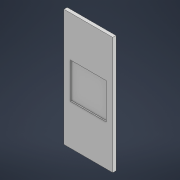
# Autodesk Inventor part: Shoulder_Cube_TestFit_V1
Saved by Autodesk Inventor 2022 (Build 260153000, 153)
## iProperties
Created: 2023-05-16
Part Number: Shoulder_Cube_TestFit_V1
Material: Generic
Document SubType Name: Modeling
Designer: Karl Spiteri
Density: 1 g/cm^3
Appearance: Default
Author: Karl Spiteri
Autodesk Inventor part; units mm, degrees
ref_plane "YZ Plane" through (0, 0, 0) normal (1, 0, 0) x (0, 1, 0)
ref_plane "XZ Plane" through (0, 0, 0) normal (0, 1, 0) x (-1, 0, 0)
ref_plane "XY Plane" through (0, 0, 0) normal (0, 0, 1) x (1, 0, 0)
sketch "Sketch1" plane through (0, 0, 0) normal (0, 0, 1) x (1, 0, 0)
  line L0 (0, 0) -> (-75, 0)
  line L1 (-75, 0) -> (-75, 180)
  line L2 (-75, 180) -> (0, 180)
  line L3 (0, 180) -> (0, 0)
  line L4 (-65, 170) -> (-10, 170)
  line L5 (-10, 10) -> (-65, 10)
  line L6 (-65, 10) -> (-65, 85)
  line L7 (-65, 95) -> (-65, 170)
  line L8 (-10, 170) -> (-10, 95)
  line L9 (-10, 85) -> (-10, 10)
  line L10 (-65, 85) -> (-65, 95)
  line L11 (-10, 95) -> (-10, 85)
  point P0 (-65, 90)
  point P1 (-10, 90)
  dimension "d35" = 75
  dimension "d36" = 180
  dimension "d37" = 55
  dimension "d38" = 160
  constraints: 24 end point, 3 parallel, 3 perpendicular, 2 horizontal, 2 midpoint, 1 collinear, 1 vertical
  measures "d35" distance of L1.end L2.end
  measures "d36" distance of L0.end L1.end
  measures "d37" distance of L5.start L5.end
  measures "d38" distance of L4.end L5.start
extrude "Extrusion16" add sketch "Sketch1" along normal blind 1
sketch "Sketch12" plane through (0, 0, 1) normal (0, 0, 1) x (1, 0, 0)
  line L0 (0, 0) -> (0, 180) projected
  line L1 (-75, 180) -> (-75, 0) projected
  line L2 (0, 180) -> (-75, 180)
  line L3 (-75, 180) -> (-75, 0)
  line L4 (-75, 0) -> (0, 0)
  line L5 (0, 0) -> (0, 180)
  constraints: 8 end point, 2 parallel, 1 horizontal, 1 perpendicular
extrude "Extrusion17" add sketch "Sketch12" along normal blind 4
sketch "Sketch13" plane through (0, 0, 5) normal (0, 0, 1) x (1, 0, 0)
  line L0 (-10, 117.5) -> (-65, 117.5)
  line L1 (-65, 117.5) -> (-65, 62.5)
  line L2 (-65, 62.5) -> (-10, 62.5)
  line L3 (-10, 62.5) -> (-10, 117.5)
  point P0 (0, 0)
  dimension "d99" = 55
  dimension "d100" = 55
  constraints: 8 end point, 2 parallel, 1 horizontal, 1 perpendicular
  measures "d99" distance of L2.end L1.end
  measures "d100" distance of L1.end L0.end
extrude "Extrusion18" cut sketch "Sketch13" against normal blind 2
body "Solid6"
